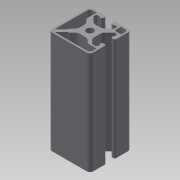
# Autodesk Inventor part: 40-4002
Saved by Autodesk Inventor 2013 (Build 170138000, 138)
## iProperties
Created: 2014-04-23
Part Number: 40-4002
Material: Generic
Document SubType Name: Modeling
Designer: Ross Bowman
Density: 1 g/cm^3
Engineer: Ross Bowman
Catalog Web Link: 8020.net
Vendor: 80/20 Inc.
Company: 80/20 Inc.
Author: Ross Bowman
Keywords: 80/20 , 8020 , T-Slot , Extrusion
Material: 6105-T5 Aluminum
Autodesk Inventor part; units mm, degrees
ref_plane "YZ Plane" through (0, 0, 0) normal (1, 0, 0) x (0, 1, 0)
ref_plane "XZ Plane" through (0, 0, 0) normal (0, 1, 0) x (-1, 0, 0)
ref_plane "XY Plane" through (0, 0, 0) normal (0, 0, 1) x (1, 0, 0)
sketch "Sketch1" plane through (0, 0, 0) normal (0, 0, 1) x (1, 0, 0)
  arc A0 (17.969, 11.935) -> (18.35, 12.316) centre (17.969, 12.316) ccw
  line L0 (13.205, 11.935) -> (17.969, 11.935)
  arc A1 (11.935, 13.205) -> (13.205, 11.935) centre (13.205, 13.205) ccw
  line L1 (11.935, 17.969) -> (11.935, 13.205)
  arc A2 (12.316, 18.35) -> (11.935, 17.969) centre (12.316, 17.969) ccw
  line L2 (15.556, 18.35) -> (12.316, 18.35)
  arc A3 (18.35, 15.556) -> (15.556, 18.35) centre (15.556, 15.556) ccw
  line L3 (18.35, 12.316) -> (18.35, 15.556)
  circle A4 centre (0, 0) radius 3.4
  arc A5 (-9.0762, -5.7416) -> (-7.685, -2.3829) centre (-12.4348, -2.3829) ccw
  line L4 (-11.6227, -8.288) -> (-9.0762, -5.7416)
  arc A6 (-11.6227, -8.288) -> (-11.8458, -8.8268) centre (-11.0838, -8.8268) ccw
  line L5 (-11.8458, -9.1968) -> (-11.8458, -8.8268)
  arc A7 (-12.069, -9.7356) -> (-11.8458, -9.1968) centre (-12.6078, -9.1968) ccw
  line L6 (-17.924, -15.5906) -> (-12.069, -9.7356)
  arc A8 (-18.35, -15.4141) -> (-17.924, -15.5906) centre (-18.1005, -15.4141) ccw
  line L7 (-18.35, 15.541) -> (-18.35, -15.4141)
  arc A9 (-15.556, 18.335) -> (-18.35, 15.541) centre (-15.556, 15.541) ccw
  line L8 (-12.316, 18.335) -> (-15.556, 18.335)
  arc A10 (-11.935, 17.954) -> (-12.316, 18.335) centre (-12.316, 17.954) ccw
  line L9 (-11.935, 9.7626) -> (-11.935, 17.954)
  arc A11 (-11.935, 9.7626) -> (-11.0051, 7.5175) centre (-8.76, 9.7626) ccw
  line L10 (-9.0762, 5.5886) -> (-11.0051, 7.5175)
  arc A12 (-7.685, 2.23) -> (-9.0762, 5.5886) centre (-12.4348, 2.23) ccw
  line L11 (-7.685, -2.3829) -> (-7.685, 2.23)
  line L12 (-15.4141, -18.35) -> (15.556, -18.35)
  arc A13 (-15.5906, -17.924) -> (-15.4141, -18.35) centre (-15.4141, -18.1005) ccw
  line L13 (-9.8056, -12.139) -> (-15.5906, -17.924)
  arc A14 (-9.2667, -11.9158) -> (-9.8056, -12.139) centre (-9.2667, -12.6778) ccw
  line L14 (-8.8204, -11.9158) -> (-9.2667, -11.9158)
  arc A15 (-8.8204, -11.9158) -> (-8.2816, -11.6926) centre (-8.8204, -11.1538) ccw
  line L15 (-5.6501, -9.0612) -> (-8.2816, -11.6926)
  arc A16 (-2.2915, -7.67) -> (-5.6501, -9.0612) centre (-2.2915, -12.4198) ccw
  line L16 (3.3048, -7.67) -> (-2.2915, -7.67)
  arc A17 (6.6634, -9.0612) -> (3.3048, -7.67) centre (3.3048, -12.4198) ccw
  line L17 (8.6072, -11.0051) -> (6.6634, -9.0612)
  arc A18 (8.6072, -11.0051) -> (10.8523, -11.935) centre (10.8523, -8.76) ccw
  line L18 (17.8551, -11.935) -> (10.8523, -11.935)
  arc A19 (18.35, -12.4299) -> (17.8551, -11.935) centre (17.8551, -12.4299) ccw
  line L19 (18.35, -15.556) -> (18.35, -12.4299)
  arc A20 (15.556, -18.35) -> (18.35, -15.556) centre (15.556, -15.556) ccw
  line L20 (-16.825, -20) -> (16.825, -20)
  arc A21 (16.825, -20) -> (20, -16.825) centre (16.825, -16.825) ccw
  line L21 (20, -16.825) -> (20, -5.6348)
  arc A22 (20, -5.6348) -> (18.4252, -4.06) centre (18.4252, -5.6348) ccw
  line L22 (18.4252, -4.06) -> (17.5148, -4.06)
  arc A23 (17.5148, -4.06) -> (15.94, -5.6348) centre (17.5148, -5.6348) ccw
  line L23 (15.94, -5.6348) -> (15.94, -6.8785)
  line L24 (15.94, -6.8785) -> (16.7025, -6.8785)
  line L25 (16.7025, -6.8785) -> (16.7025, -9.015)
  arc A24 (15.4325, -10.285) -> (16.7025, -9.015) centre (15.4325, -9.015) ccw
  line L26 (15.4325, -10.285) -> (12.4956, -10.285)
  arc A25 (11.867, -10.0246) -> (12.4956, -10.285) centre (12.4956, -9.396) ccw
  line L27 (11.867, -10.0246) -> (9.0762, -7.2338)
  arc A26 (7.685, -3.8752) -> (9.0762, -7.2338) centre (12.4348, -3.8752) ccw
  line L28 (7.685, -3.8752) -> (7.685, 2.341)
  arc A27 (9.0762, 5.6996) -> (7.685, 2.341) centre (12.4348, 2.341) ccw
  line L29 (9.0762, 5.6996) -> (13.4012, 10.0246)
  arc A28 (14.0298, 10.285) -> (13.4012, 10.0246) centre (14.0298, 9.396) ccw
  line L30 (14.0298, 10.285) -> (15.432, 10.285)
  arc A29 (16.702, 9.015) -> (15.432, 10.285) centre (15.432, 9.015) ccw
  line L31 (16.702, 9.015) -> (16.702, 6.8785)
  line L32 (16.702, 6.8785) -> (15.94, 6.8785)
  line L33 (15.94, 6.8785) -> (15.94, 5.6348)
  arc A30 (15.94, 5.6348) -> (17.5148, 4.06) centre (17.5148, 5.6348) ccw
  line L34 (17.5148, 4.06) -> (18.4252, 4.06)
  arc A31 (18.4252, 4.06) -> (20, 5.6348) centre (18.4252, 5.6348) ccw
  line L35 (20, 5.6348) -> (20, 16.825)
  arc A32 (20, 16.825) -> (16.825, 20) centre (16.825, 16.825) ccw
  line L36 (16.825, 20) -> (5.6348, 20)
  arc A33 (5.6348, 20) -> (4.06, 18.4252) centre (5.6348, 18.4252) ccw
  line L37 (4.06, 18.4252) -> (4.06, 17.5148)
  arc A34 (4.06, 17.5148) -> (5.6348, 15.94) centre (5.6348, 17.5148) ccw
  line L38 (5.6348, 15.94) -> (6.8785, 15.94)
  line L39 (6.8785, 15.94) -> (6.8785, 16.7025)
  line L40 (6.8785, 16.7025) -> (9.015, 16.7025)
  arc A35 (10.285, 15.4325) -> (9.015, 16.7025) centre (9.015, 15.4325) ccw
  line L41 (10.285, 15.4325) -> (10.285, 14.0298)
  arc A36 (10.0246, 13.4012) -> (10.285, 14.0298) centre (9.396, 14.0298) ccw
  line L42 (10.0246, 13.4012) -> (5.7146, 9.0912)
  arc A37 (2.356, 7.7) -> (5.7146, 9.0912) centre (2.356, 12.4498) ccw
  line L43 (2.356, 7.7) -> (-2.356, 7.7)
  arc A38 (-5.7146, 9.0912) -> (-2.356, 7.7) centre (-2.356, 12.4498) ccw
  line L44 (-5.7146, 9.0912) -> (-10.0246, 13.4012)
  arc A39 (-10.285, 14.0298) -> (-10.0246, 13.4012) centre (-9.396, 14.0298) ccw
  line L45 (-10.285, 14.0298) -> (-10.285, 15.4325)
  arc A40 (-9.015, 16.7025) -> (-10.285, 15.4325) centre (-9.015, 15.4325) ccw
  line L46 (-9.015, 16.7025) -> (-6.8785, 16.7025)
  line L47 (-6.8785, 16.7025) -> (-6.8785, 15.94)
  line L48 (-6.8785, 15.94) -> (-5.6348, 15.94)
  arc A41 (-5.6348, 15.94) -> (-4.06, 17.5148) centre (-5.6348, 17.5148) ccw
  line L49 (-4.06, 17.5148) -> (-4.06, 18.4252)
  arc A42 (-4.06, 18.4252) -> (-5.6348, 20) centre (-5.6348, 18.4252) ccw
  line L50 (-5.6348, 20) -> (-16.825, 20)
  arc A43 (-16.825, 20) -> (-20, 16.825) centre (-16.825, 16.825) ccw
  line L51 (-20, 16.825) -> (-20, -16.825)
  arc A44 (-20, -16.825) -> (-16.825, -20) centre (-16.825, -16.825) ccw
  constraints: 104 end point, 88 point on circle, 45 centre point
extrude "Extrusion1" add sketch "Sketch1" against normal blind 100
body "Solid1"
